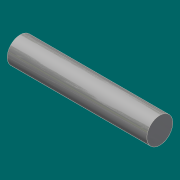
# Autodesk Inventor part: A1-19027-400-14 Plug shaft
Saved by Autodesk Inventor 2017.3 (Build 213257000, 257)
## iProperties
Created: 2019-08-16
Part Number: A1-19027-400-14 Plug shaft
Material: Steel, Mild
Document SubType Name: Modeling
Designer: GVD
Density: 7.85 g/cm^3
Appearance: Steel
Mass: 599.638 g
Surface Area: 130.969 cm^2
Volume: 76.387 cm^3
Description: Ø1" x 5 3/8" ROUND BAR, A36
Author: GVD
Autodesk Inventor part; units mm, degrees
ref_plane "YZ Plane" through (0, 0, 0) normal (1, 0, 0) x (0, 1, 0)
ref_plane "XZ Plane" through (0, 0, 0) normal (0, 1, 0) x (-1, 0, 0)
ref_plane "XY Plane" through (0, 0, 0) normal (0, 0, 1) x (1, 0, 0)
sketch "Sketch1" plane through (0, 0, 0) normal (0, 0, 1) x (1, 0, 0)
  line L0 (0, 0) -> (136.525, 0)
  line L1 (136.525, 0) -> (136.525, 12.7)
  line L2 (136.525, 12.7) -> (0, 12.7)
  line L3 (0, 12.7) -> (0, 0)
  dimension "d0" = 136.525
  dimension "d1" = 25.4
  constraints: 8 end point, 3 perpendicular, 1 horizontal
  measures "d0" distance of L0.start L0.end
  measures "d1" diameter of L2 L0
revolve "Revolution1" add sketch "Sketch1" angle 360 about axis through (0, 0, 0) along (1, 0, 0)
body "Solid1"
